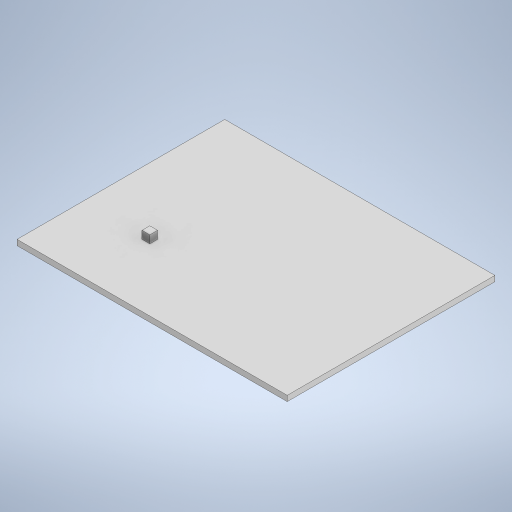
# Autodesk Inventor part: Cabinet - left
Saved by Autodesk Inventor 2024.3 (Build 283343000, 343)
## iProperties
Created: 2025-03-26
Part Number: Cabinet - left
Material: Všeobecné
Document SubType Name: Modeling
Designer: admin
Density: 1 g/cm^3
Appearance: Výchozí
Author: admin
Autodesk Inventor part; units mm, degrees
ref_plane "YZ Plane" through (0, 0, 0) normal (1, 0, 0) x (0, 1, 0)
ref_plane "XZ Plane" through (0, 0, 0) normal (0, 1, 0) x (-1, 0, 0)
ref_plane "XY Plane" through (0, 0, 0) normal (0, 0, 1) x (1, 0, 0)
sketch "Náčrt1" plane through (0, 0, 0) normal (0, 1, 0) x (-1, 0, 0)
  line L0 (0, -93.1) -> (0, 93.1) projected
  line L1 (-121.1, 0) -> (121.1, 0) projected
  line L2 (86.5, 66.5) -> (-86.5, 66.5)
  line L3 (-86.5, 66.5) -> (-86.5, -66.5)
  line L4 (-86.5, -66.5) -> (86.5, -66.5)
  line L5 (86.5, -66.5) -> (86.5, 66.5)
  point P0 (0, 0)
  dimension "d0" = 133
  dimension "d1" = 173
  constraints: 8 end point, 2 parallel, 1 horizontal, 1 perpendicular, 2 other
  measures "d0" distance of L2.end L3.end
  measures "d1" distance of L3.end L4.end
extrude "Vysunutí1" add sketch "Náčrt1" along normal mid plane 3.5
sketch "Náčrt2" plane through (0, 1.75, 0) normal (0, 1, 0) x (1, 0, 0)
  line L0 (-46.5, -26.5) -> (-41.5, -26.5)
  line L1 (-41.5, -26.5) -> (-41.5, -21.5)
  line L2 (-41.5, -21.5) -> (-46.5, -21.5)
  line L3 (-46.5, -21.5) -> (-46.5, -26.5)
  line L4 (-86.5, -66.5) -> (86.5, -66.5) projected
  line L5 (-86.5, 66.5) -> (-86.5, -66.5) projected
  point P0 (0, 0)
  dimension "d4" = 5
  dimension "d5" = 5
  dimension "d6" = 40
  dimension "d7" = 40
  constraints: 8 end point, 2 parallel, 1 horizontal, 1 perpendicular
  measures "d4" distance of L0.end L1.end
  measures "d5" distance of L1.end L2.end
  measures "d6" distance between parallel lines of L4 L0
  measures "d7" distance between parallel lines of L5 L3
extrude "Vysunutí2" add sketch "Náčrt2" along normal blind 5
